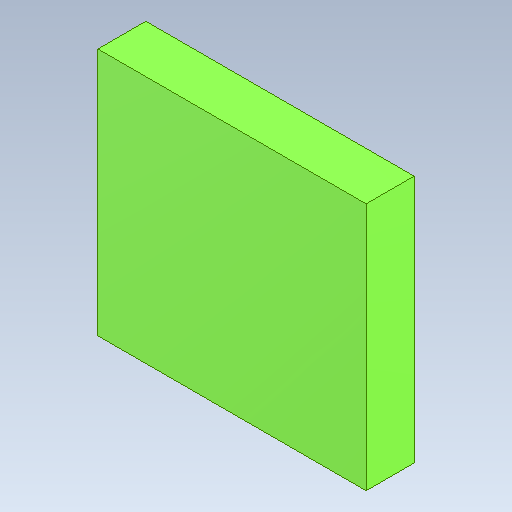
# Autodesk Inventor part: A4950ELJTR-T
Saved by Autodesk Inventor 2020 (Build 240168000, 168)
## iProperties
Created: 2019-08-29
Part Number: A4950ELJTR-T
Material: Generic
Document SubType Name: Modeling
Designer: psrob
Density: 1 g/cm^3
Appearance: SOIC8TP, A4950ELJTR-T
Author: psrob
Autodesk Inventor part; units mm, degrees
ref_plane "YZ Plane" through (0, 0, 0) normal (1, 0, 0) x (0, 1, 0)
ref_plane "XZ Plane" through (0, 0, 0) normal (0, 1, 0) x (-1, 0, 0)
ref_plane "XY Plane" through (0, 0, 0) normal (0, 0, 1) x (1, 0, 0)
sketch "SOIC8TP, A4950ELJTR-T_48" plane through (0, 0, 0) normal (0, 0, 1) x (1, 0, 0)
  line L0 (-2.7995, 2.6416) -> (2.7951, 2.6416)
  line L1 (2.7951, 2.6416) -> (2.7951, -2.54)
  line L2 (2.7951, -2.54) -> (-2.7995, -2.54)
  line L3 (-2.7995, -2.54) -> (-2.7995, 2.6416)
  constraints: 8 end point
extrude "Extrusion1" add sketch "SOIC8TP, A4950ELJTR-T_48" along normal blind 1
body "Solid1"
